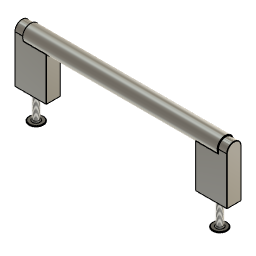
Hafele Handle 115.70 (Autodesk Fusion 360 design; units mm, degrees)
description: Hafele Handle
part number: 115.70.xx
description: Screw M4
part number: M4
Autodesk Fusion 360 part; units mm, degrees
note: some values were not read from the file. Chosen so that the rebuilt part matches the saved one: which bodies a step acts on; how an offset face is resized. Set by a fixed rule: the direction of a hole.
sketch "Control" plane through (0, 0, 0) normal (0, 0, 1) x (1, 0, 0)
  line L0 (200, -350) -> (-200, -350)
  line L1 (-200, -350) -> (-200, 350)
  line L2 (-200, 350) -> (200, 350)
  line L3 (200, 350) -> (200, -350)
  line L4 (200, -350) -> (-200, 350) construction
  line L5 (-200, -350) -> (200, 350) construction
  point P0 (0, 285)
  dimension "d7" = 700
  dimension "d8" = 400
  dimension "d9" = 200
  dimension "d100" = 65
  constraint horizontal L0
  constraint perpendicular L0 L1
  constraint parallel L0 L2
  constraint parallel L1 L3
  constraint coincident L4 origin
  constraint coincident L5 origin
  measures "d7" distance of L0.end L1.end
  measures "d8" distance of L1 L3
  measures "d9" distance of L1 P0
  measures "d100" vertical distance of L1.end P0
sketch "Handle" plane through (0, 0, 0) normal (0, 0, 1) x (1, 0, 0)
  line L0 (74, 280) -> (-74, 280)
  line L1 (-74, 280) -> (-74, 290)
  line L2 (-74, 290) -> (74, 290)
  line L3 (74, 290) -> (74, 280)
  line L4 (74, 280) -> (-74, 290) construction
  line L5 (-74, 280) -> (74, 290) construction
  point P0 (0, 285)
  point P1 (0, 285)
  dimension "d12" = 10
  dimension "d13" = 148
  constraint horizontal L0
  constraint perpendicular L0 L1
  constraint parallel L0 L2
  constraint parallel L1 L3
  constraint coincident L4 P1
  constraint coincident L5 P1
  constraint coincident P0 P1
  measures "d12" distance of L0.end L1.end
  measures "d13" distance of L1 L3
ref_plane "WorkPlane1" through (0, 285, 0) normal (0, 1, 0) x (0, 0, 1)
ref_plane "WorkPlane2" through (0, 0, 0) normal (1, 0, 0) x (0, 1, 0)
sketch "Sketch3" plane through (0, 0, 0) normal (1, 0, 0) x (0, 1, 0)
  line L0 (280, 0) -> (290, 0)
  line L1 (290, 0) -> (290, 38)
  line L2 (290, 38) -> (280, 38)
  line L3 (280, 38) -> (280, 0)
  line L4 (280, 0) -> (290, 38) construction
  line L5 (290, 0) -> (280, 38) construction
  line L6 (350, 0) -> (-350, 0)
  point P0 (285, 19)
  point P1 (285, 0)
  dimension "d16" = 10
  dimension "d17" = 38
  constraint horizontal L0
  constraint perpendicular L0 L1
  constraint parallel L0 L2
  constraint parallel L1 L3
  constraint coincident L4 P0
  constraint coincident L5 P0
  constraint vertical P0 P1
  constraint collinear L0 L6
  measures "d16" distance of L1.end L2.end
  measures "d17" distance of L0 L2
extrude "Extrude1" add sketch "Sketch3" along normal mid plane 148 makes body 1 in component "Hafele Handle 115.70"
sketch "Sketch1" plane through (0, 290, 0) normal (0, 1, 0) x (-1, 0, 0) in component "Hafele Handle 115.70"
  line L0 (74, 38) -> (-74, 38)
  line L1 (-74, 38) -> (-74, 0)
  line L2 (-74, 0) -> (74, 0)
  line L3 (74, 0) -> (74, 38)
  line L4 (-52, 38) -> (52, 38)
  line L5 (52, 38) -> (52, 0)
  line L6 (52, 0) -> (-52, 0)
  line L7 (-52, 0) -> (-52, 38)
  line L8 (-52, 38) -> (52, 0) construction
  line L9 (52, 38) -> (-52, 0) construction
  line L10 (200, 0) -> (-200, 0)
  point P0 (0, 19)
  dimension "d20" = 22
  constraint horizontal L4
  constraint perpendicular L4 L5
  constraint parallel L4 L6
  constraint parallel L5 L7
  constraint coincident L8 P0
  constraint coincident L9 P0
  constraint vertical P0 origin
  constraint collinear L6 L10
  constraint collinear L0 L4
  measures "d20" distance of L3 L5
extrude "Extrude2" cut sketch "Sketch1" against normal up to surface (10 mm away) contours L0 L2 L4 L5 L6 L7 L10 bodies 1 makes body 2 at (59.3333, 290, 25.3333) in component "Hafele Handle 115.70"
fillet "Fillet1" radius 5 4 edges at (-63, 290, 38) (-63, 280, 38) (63, 290, 38) (63, 280, 38) on bodies 1 2 in component "Hafele Handle 115.70"
sketch "Sketch2" plane through (0, 285, 0) normal (0, 1, 0) x (1, 0, 0) in component "Hafele Handle 115.70"
  line L0 (68, -38.6667) -> (-68, -38.6667)
  line L1 (-68, -38.6667) -> (-68, -33)
  line L2 (-68, -33) -> (68, -33)
  line L3 (68, -33) -> (68, -38.6667)
  line L4 (68, -38.6667) -> (-68, -33) construction
  line L5 (-68, -38.6667) -> (68, -33) construction
  line L6 (-74, 0) -> (-74, -33)
  line L7 (41, -33) -> (85, -33)
  line L8 (-52, -33) -> (-52, -38)
  line L9 (-52, -33) -> (-74, -33)
  line L10 (-74, -38) -> (-74, -33)
  line L11 (-74, -33) -> (-52, -33)
  point P0 (0, -35.8333)
  dimension "d25" = 6
  constraint horizontal L0
  constraint perpendicular L0 L1
  constraint parallel L0 L2
  constraint parallel L1 L3
  constraint coincident L4 P0
  constraint coincident L5 P0
  constraint vertical P0 origin
  constraint collinear L2 L7
  constraint coincident L5 L8.end
  measures "d25" distance of L1 L6
revolve "Revolve1" cut sketch "Sketch2" angle 360 about axis through (41, 285, 33) along (1, 0, 0) bodies 1 2 in component "Hafele Handle 115.70"
revolve "Revolve2" add sketch "Sketch2" angle 360 about axis through (41, 285, 33) along (1, 0, 0) separate body makes body 3 in component "Hafele Handle 115.70"
chamfer "Chamfer1" distance 0.2 angle 45 10 edges at (52, 290, 15.1667) (74, 290, 16.5) (74, 285, 38) (74, 280, 16.5) (52, 280, 15.1667) (-52, 290, 15.1667) (-52, 280, 15.1667) (-74, 290, 16.5) (-74, 280, 16.5) (-74, 285, 38) on bodies 1 2 in component "Hafele Handle 115.70"
fillet "Fillet2" radius 0.1 4 edges at (-60.1, 290, 30.3333) (-60.1, 280, 30.3333) (60.1, 290, 30.3333) (60.1, 280, 30.3333) on bodies 1 2 in component "Hafele Handle 115.70"
fillet "Fillet2" radius 0.1 6 edges at (-68, 280, 31.6667) (-68, 285, 38) (-68, 290, 31.6667) (68, 290, 31.6667) (68, 285, 38) (68, 280, 31.6667) on bodies 1 2 in component "Hafele Handle 115.70"
chamfer "Chamfer2" distance 0.2 angle 45 2 edges at (-68, 282.9508, 27.7168) (68, 282.9508, 27.7168) on bodies 3 in component "Hafele Handle 115.70"
sketch "Sketch3 (2)" plane through (0, 0, 0) normal (0, 0, 1) x (1, 0, 0) in component "Hafele Handle 115.70"
  line L0 (64, 285) -> (-64, 285) construction
  point P0 (74, 280)
  point P1 (-74, 280)
  point P2 (0, 285)
  dimension "d34" = 10
  dimension "d35" = 10
  constraint horizontal L0
  constraint coincident L0 P2
  measures "d34" horizontal distance of L0.start P0
  measures "d35" horizontal distance of L0.end P1
hole "Hole1" at (64, 285, 0) at (-64, 285, 0) direction (0, 0, 1) diameter 3.332 depth 20 tip angle 118 countersink diameter 4.5 countersink angle 90 bodies 1 2 in component "Hafele Handle 115.70"
thread "Thread1" "ISO Metric profile 4.0 M4x0.7 6H" in component "Hafele Handle 115.70"
ref_plane "WorkPlane3" through (-64, 285, 10.292) normal (-1, 0, 0) x (0, 0, 1)
sketch "Sketch4" plane through (-64, 285, 10.292) normal (-1, 0, 0) x (0, 1, 0)
  line L0 (0, 19.416) -> (0, -19.416)
  line L1 (2.5, 28.292) -> (0, 28.292)
  line L2 (0, 28.292) -> (0, 10.292)
  line L3 (0, 10.292) -> (2.5, 10.292)
  line L4 (2.5, 10.292) -> (2.5, 28.292)
  line L5 (4.8, 10.292) -> (-4.8, 10.292)
  dimension "d47" = 5
  dimension "d48" = 18
  constraint horizontal L1
  constraint vertical L2
  constraint horizontal L3
  constraint vertical L4
  constraint coincident L0 L2.end
  constraint collinear L3 L5
  measures "d48" distance of L1 L3
revolve "Revolve1'" add sketch "Sketch4" angle 360 about axis through (-64, 285, -9.124) along (0, 0, 1) separate body makes body 4 in component "Screw M4"
sketch "Sketch1 (2)" plane through (-64, 285, 10.292) normal (-1, 0, 0) x (0, 1, 0) in component "Screw M4"
  line L0 (0, 19.416) -> (0, -19.416)
  line L1 (2, 28.292) -> (0, 28.292)
  line L2 (0, 28.292) -> (0, 8.292)
  line L3 (0, 8.292) -> (2, 8.292)
  line L4 (2, 8.292) -> (2, 28.292)
  line L5 (-2.5, 28.292) -> (2.5, 28.292)
  line L6 (2, 28.292) -> (1.75, 28.292)
  line L7 (1.75, 28.292) -> (1.75, 27.692)
  line L8 (1.75, 27.692) -> (2, 27.692)
  line L9 (2, 27.692) -> (2, 28.292)
  line L10 (5, 29.092) -> (0, 29.092)
  line L11 (0, 29.092) -> (0, 28.292)
  line L12 (0, 28.292) -> (5, 28.292)
  line L13 (5, 28.292) -> (5, 29.092)
  arc A0 (4, 29.092) -> (0, 30.592) centre (0, 24.5087) ccw
  line L14 (0, 30.592) -> (0, 29.092)
  point P0 (4, 29.092)
  dimension "d59" = 4
  dimension "d60" = 20
  dimension "d61" = 0.25
  dimension "d62" = 0.6
  dimension "d63" = 10
  dimension "d64" = 0.8
  dimension "d65" = 1
  dimension "d66" = 1.5
  constraint horizontal L1
  constraint vertical L2
  constraint horizontal L3
  constraint vertical L4
  constraint collinear L0 L2
  constraint collinear L1 L5
  constraint horizontal L6
  constraint vertical L7
  constraint horizontal L8
  constraint vertical L9
  constraint horizontal L10
  constraint vertical L11
  constraint horizontal L12
  constraint vertical L13
  constraint collinear L2 L11
  constraint collinear L1 L12
  constraint coincident L10 P0
  constraint coincident P0 A0.start
  constraint coincident L2 A0.centre
  constraint vertical A0.end A0.centre
  measures "d60" distance of L1.start L3.end
  measures "d61" distance of L1.start L6.end
  measures "d62" distance of L1.start L8.end
  measures "d64" distance of L10 L12
  measures "d65" distance of L13 P0
  measures "d66" distance of L10 A0.end
revolve "Revolve2'" add sketch "Sketch1 (2)" angle 360 about axis through (-64, 285, -9.124) along (0, 0, 1) separate body contours L0 L1 L2 L3 L4 L5 L7 L8 L12 | L1 L5 L6 L10 L11 L12 L13 | L10 A0 L14 makes body 5 in component "Screw M4"
chamfer "Chamfer1'" distance 0.5 angle 45 1 edges at (-65.8647, 284.2768, 2) on bodies 5 in component "Screw M4"
ref_plane "WorkPlane1" through (-64, 285, -20.3) normal (0, 0, -1) x (-1, 0, 0) in component "Screw M4"
thread "Thread1'" "ISO Metric profile 4.0 M4x0.7 6g" major diameter 3.908 minor diameter 3.111 pitch 0.7 angle 60 resizes the face on face at (-64.7769, 286.843, -4.8) on bodies 5 in component "Screw M4"
chamfer "Chamfer3" distance 0.2 angle 45 1 edges at (-63.2934, 283.1782, -17.4) on bodies 5 in component "Screw M4"
fillet "Fillet1'" radius 1 1 edges at (-65.6316, 284.3672, -18) on bodies 5 in component "Screw M4"
fillet "Fillet2'" radius 0.3 2 edges at (-68.6616, 283.1919, -18) (-68.6616, 283.1919, -18.8) on bodies 5 in component "Screw M4"
sketch "Sketch3 (3)" plane through (-64, 285, 10.292) normal (-1, 0, 0) x (0, 1, 0) in component "Screw M4"
  line L0 (0, 19.416) -> (0, -19.416)
  line L1 (1.5, 8.292) -> (0, 8.292)
  line L2 (0, 8.292) -> (0, 6.792)
  line L3 (0, 6.792) -> (1.5, 6.792)
  line L4 (1.5, 6.792) -> (1.5, 8.292)
  line L5 (1.5, 8.292) -> (-1.5, 8.292)
  line L6 (1.5, 6.792) -> (1.954, 6.338)
  line L7 (1.954, 6.338) -> (1.954, 3.746)
  line L8 (1.954, 3.746) -> (1.5, 3.292)
  line L9 (1.5, 3.292) -> (0, 3.292)
  line L10 (0, 3.292) -> (0, 6.792)
  line L11 (-1.954, 8.746) -> (1.954, 8.746)
  dimension "d83" = 45
  dimension "d84" = 45
  dimension "LL" = 5
  dimension "d86" = 1.5
  constraint horizontal L1
  constraint vertical L2
  constraint horizontal L3
  constraint vertical L4
  constraint collinear L0 L2
  constraint collinear L1 L5
  constraint perpendicular L3 L7
  constraint perpendicular L7 L9
  constraint perpendicular L3 L10
  constraint vertical L3.end L8.end
  constraint vertical L6.end L11.end
  constraint vertical L3.end L1.start
  measures "d83" angle of L4 L6
  measures "d84" angle of L4 L8
  measures "LL" distance of L1 L9
  measures "d86" distance of L1.start L3.end
revolve "Revolve3" add sketch "Sketch3 (3)" angle 360 about axis through (-64, 285, -9.124) along (0, 0, 1) bodies 5 in component "Screw M4"
thread "Thread2" "ISO Metric profile 4.0 M4x0.7 6g" in component "Screw M4"
pattern_linear "R-Pattern1" [suppressed] in component "Screw M4"
sketch "Sketch4 (2)" plane through (0, 0, -18.8) normal (0, 0, -1) x (1, 0, 0) in component "Screw M4"
  circle A0 centre (-64, -285) radius 4
  circle A1 centre (-64, -285) radius 4.7
  circle A2 centre (-64, -285) radius 4.7
  line L0 (-68.25, -284.7) -> (-59.75, -284.7)
  line L1 (-59.75, -284.7) -> (-59.75, -285.3)
  line L2 (-59.75, -285.3) -> (-68.25, -285.3)
  line L3 (-68.25, -285.3) -> (-68.25, -284.7)
  line L4 (-68.25, -284.7) -> (-59.75, -285.3) construction
  line L5 (-59.75, -284.7) -> (-68.25, -285.3) construction
  line L6 (-64.3, -282) -> (-63.7, -282)
  line L7 (-63.7, -282) -> (-63.7, -288)
  line L8 (-63.7, -288) -> (-64.3, -288)
  line L9 (-64.3, -288) -> (-64.3, -282)
  line L10 (-64.3, -282) -> (-63.7, -288) construction
  line L11 (-63.7, -282) -> (-64.3, -288) construction
  point P0 (-64, -285)
  point P1 (-64, -285)
  dimension "d101" = 8.5
  dimension "d102" = 0.6
  dimension "d103" = 0.6
  dimension "d104" = 6
  constraint horizontal L0
  constraint perpendicular L0 L1
  constraint parallel L0 L2
  constraint parallel L1 L3
  constraint coincident L4 P1
  constraint coincident L5 P1
  constraint coincident P1 P0
  constraint horizontal L6
  constraint perpendicular L6 L7
  constraint parallel L6 L8
  constraint parallel L7 L9
  constraint coincident L10 P1
  constraint coincident L11 P1
  measures "d101" distance of L1.end L2.end
  measures "d102" distance of L0.end L1.end
  measures "d103" distance of L7.end L8.end
  measures "d104" distance of L6.end L7.end
extrude "Extrude2'" cut sketch "Sketch4 (2)" along normal blind 1.5 draft 10 contours A0 L0 L2 L7 | A0 L0 L1 L2 | A0 L0 L2 L9 | A0 L0 L2 L3 | L0 L2 L7 L9 | L0 L6 L7 L9 | L2 L7 L8 L9 bodies 5 in component "Screw M4"
chamfer "Chamfer4" distance 0.5 angle 45 4 edges at (-63.5722, 285.4278, -19.5245) (-64.4278, 285.4278, -19.5245) (-63.5722, 284.5722, -19.5245) (-64.4278, 284.5722, -19.5245) on bodies 5 in component "Screw M4"
component "Hafele Handle 115.70" placed x (1, 0, 0) y (0, 1, 0) z (0, 0, 1) at (0, 0, 0)
component "Screw M4" placed x (1, 0, 0) y (0, 1, 0) z (0, 0, 1) at (0, 0, 0)
component "Screw M4" placed x (1, 0, 0) y (0, 1, 0) z (0, 0, 1) at (128, 0, 0)
equation "FacadeWidth = 400 mm"
equation "FacadeHeight = 700 mm"
equation "HandleHorPos = FacadeWidth / 2"
equation "HandleVertPos = 65 mm"
equation "d7 = FacadeHeight"
equation "d8 = FacadeWidth"
equation "d9 = HandleHorPos"
equation "HandleLength = 148 mm" comment "Possible lengths: 148; 180; 212; 244; 340"
equation "d13 = HandleLength"
equation "d18 = HandleLength"
equation "FacadeThickness = 18 mm"
equation "d48 = FacadeThickness"
equation "d90 = LL"
equation "d100 = HandleVertPos"
named bodies: "Screw Hole", "Screw"
